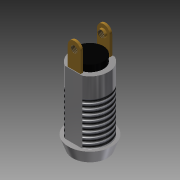
# Autodesk Inventor part: KeySwitchBody
Saved by Autodesk Inventor 2016 (Build 200138000, 138)
## iProperties
Created: 2014-09-27
Part Number: KeySwitchBody
Material: Steel, Alloy
Document SubType Name: Modeling
Designer: Jack
Density: 7.73 g/cm^3
Appearance: Semi-Polished
Mass: 83.2063 g
Surface Area: 38.3023 cm^2
Volume: 10.7641 cm^3
Author: Jack
Autodesk Inventor part; units mm, degrees
ref_plane "YZ Plane" through (0, 0, 0) normal (1, 0, 0) x (0, 1, 0)
ref_plane "XZ Plane" through (0, 0, 0) normal (0, 1, 0) x (-1, 0, 0)
sketch "Sketch1" plane through (0, 0, 0) normal (0, 0, 1) x (1, 0, 0)
  circle A0 centre (0, 0) radius 9.375
  dimension "d0" = 18.75
  constraints: 1 centre point, 1 coincident
  measures "d0" diameter of A0
extrude "Extrusion1" add sketch "Sketch1" along normal blind 32
sketch "Sketch2" plane through (0, 0, 32) normal (0, 0, 1) x (1, 0, 0)
  circle A0 centre (0, 0) radius 9.375 projected
  circle A1 centre (0, 0) radius 6.8
  dimension "d3" = 13.6
  constraints: 1 centre point, 1 coincident
  measures "d3" diameter of A1
extrude "Extrusion2" add sketch "Sketch2" along normal blind 3.3 contours A1
sketch "Sketch3" plane through (0, 0, 32) normal (0, 0, 1) x (1, 0, 0)
  circle A0 centre (0, 0) radius 6.8 projected
  line L0 (-3.25, 8) -> (3.25, 8)
  line L1 (-3.25, -8) -> (3.25, -8)
  line L2 (-3.25, 8) -> (-3.25, 6.8)
  line L3 (-3.25, 6.8) -> (3.25, 6.8)
  line L4 (3.25, 6.8) -> (3.25, 8)
  line L5 (-3.25, -8) -> (-3.25, -6.8)
  line L6 (-3.25, -6.8) -> (3.25, -6.8)
  line L7 (3.25, -6.8) -> (3.25, -8)
  dimension "d6" = 6.5
  dimension "d7" = 6.5
  dimension "d8" = 3.25
  dimension "d9" = 3.25
  dimension "d10" = 1.2
  dimension "d11" = 1.2
  dimension "d12" = 16
  dimension "d13" = 8
  constraints: 16 end point, 4 perpendicular, 2 horizontal, 2 vertical
  measures "d6" distance of L1.start L1.end
  measures "d7" distance of L0.start L0.end
  measures "d8" horizontal distance of A0.centre L1.end
  measures "d9" horizontal distance of L0.end A0.centre
  measures "d10" distance of L0.start L2.end
  measures "d11" distance of L1.start L5.end
  measures "d12" distance between parallel lines of L1 L0
  measures "d13" distance from line of A0.centre L0
extrude "Extrusion3" add sketch "Sketch3" along normal blind 13 contours L6 L7 L1 L5 | L3 L2 L0 L4
sketch "Sketch4" plane through (-3.25, -8, 32) normal (0, -1, 0) x (1, 0, 0)
  line L0 (6.5, 0) -> (6.5, 13) projected
  line L1 (0, 13) -> (6.5, 13) projected
  circle A0 centre (3.25, 9.2) radius 1.7
  point P0 (3.25, -32)
  dimension "d16" = 3.4
  dimension "d17" = 3.25
  dimension "d18" = 3.8
  constraints: 1 centre point
  measures "d16" diameter of A0
  measures "d17" distance from line of L0 A0.centre
  measures "d18" distance from line of L1 A0.centre
extrude "Extrusion4" cut sketch "Sketch4" against normal up to surface (16 mm away)
fillet "Fillet1" radius 3.25 4 edges at (-3.25, -7.4, 45) (3.25, -7.4, 45) (-3.25, 7.4, 45) (3.25, 7.4, 45)
sketch "Sketch5" plane through (-3.25, 6.8, 32) normal (0, -1, 0) x (1, 0, 0)
  circle A0 centre (3.25, 9.2) radius 1.7 projected
  circle A1 centre (3.25, 9.2) radius 1.95
  point P0 (3.25, -32)
  dimension "d22" = 3.9
  constraints: 1 centre point, 1 coincident
  measures "d22" diameter of A1
extrude "Extrusion5" add sketch "Sketch5" along normal blind 1.2
sketch "Sketch6" plane through (0, -6.8, 32) normal (0, 1, 0) x (1, 0, 0)
  circle A0 centre (0, -9.2) radius 1.7 projected
  circle A1 centre (0, -9.2) radius 1.95
  point P0 (0, 32)
  dimension "d25" = 3.9
  constraints: 1 centre point, 1 coincident
  measures "d25" diameter of A1
extrude "Extrusion6" add sketch "Sketch6" along normal blind 1.2
sketch "Sketch7" plane through (0, 0, 0) normal (0, 0, -1) x (-1, 0, 0)
  circle A0 centre (0, 0) radius 9.375 projected
  circle A1 centre (0, 0) radius 10.95
  dimension "d28" = 21.9
  constraints: 1 centre point, 1 coincident
  measures "d28" diameter of A1
ref_plane "Work Plane1" through (0, 0, -6.2) normal (0, 0, -1) x (-1, 0, 0)
sketch "Sketch8" plane through (0, 0, -6.2) normal (0, 0, -1) x (-1, 0, 0)
  circle A0 centre (0, 0) radius 9.375 projected
  circle A1 centre (0, 0) radius 8.75
  dimension "d30" = 17.5
  constraints: 1 centre point, 1 coincident
  measures "d30" diameter of A1
loft "Loft1" add profiles "Sketch7", "Sketch8" contours A0 | A1 / A1
sketch "Sketch9" plane through (0, 0, 32) normal (0, 0, 1) x (1, 0, 0)
  circle A0 centre (0, 0) radius 9.375 projected
  line L0 (-4.359, 8.3) -> (4.359, 8.3)
  line L1 (-4.359, -8.3) -> (4.359, -8.3)
  point P0 (8.3, 4.359)
  point P1 (8.3, -4.359)
  point P2 (-8.3, 4.359)
  point P3 (-8.3, -4.359)
  dimension "d51" = 16.6
  dimension "d52" = 8.3
  constraints: 4 end point, 1 horizontal, 1 parallel, 9 other
  measures "d51" distance between parallel lines of L0 L1
  measures "d52" distance from line of point (0, 0) L1
thread "Thread1" size "M20x2.5" class "6g" standard "ANSI Metric M Profile" length 22
thread "Thread2" size "M20x2.5" class "6g" standard "ANSI Metric M Profile" length 22
thread "Thread3" size "M3.5x0.6" class "6H" standard "ANSI Metric M Profile" length 10
thread "Thread4" size "M3.5x0.6" class "6H" standard "ANSI Metric M Profile" length 10
sketch "Sketch10" plane through (0, 0, -6.2) normal (0, 0, -1) x (-1, 0, 0)
  circle A0 centre (0, 0) radius 8.75 projected
  circle A1 centre (0, 0) radius 4.9
  circle A2 centre (0, 0) radius 3.8
  dimension "d47" = 9.8
  dimension "d48" = 7.6
  constraints: 2 centre point, 2 coincident
  measures "d47" diameter of A1
  measures "d48" diameter of A2
extrude "Extrusion8" cut sketch "Sketch10" against normal blind 6 contours A1
extrude "Extrusion9" cut sketch "Sketch9" against normal up to surface (32 mm away) contours L0 A0 | A0 L1
sketch "Sketch11" plane through (0, 0, -6.2) normal (0, 0, -1) x (-1, 0, 0)
  circle A0 centre (0, 0) radius 3.8 projected
  circle A1 centre (0, 0) radius 8.75 projected
  circle A2 centre (0, 0) radius 4.9 projected
  line L0 (6.1, 0.75) -> (1.7, 0.75)
  line L1 (1.7, 0.75) -> (1.7, -0.75)
  line L2 (1.7, -0.75) -> (6.1, -0.75)
  line L3 (6.1, -0.75) -> (6.1, 0.75)
  circle A3 centre (0, 0) radius 4.9 projected
  line L4 (0.75, -4.8423) -> (0.75, -6.1)
  line L5 (0.75, -6.1) -> (-0.75, -6.1)
  line L6 (-0.75, -6.1) -> (-0.75, -4.8423)
  dimension "d55" = 4.4
  dimension "d56" = 1.5
  dimension "d57" = 1.5
  dimension "d58" = 1.2
  dimension "d59" = 0.75
  dimension "d60" = 1.2
  dimension "d61" = 0.75
  constraints: 14 end point, 4 point on circle, 2 parallel, 2 perpendicular, 2 vertical, 1 horizontal
  measures "d55" distance of L2.end L1.end
  measures "d56" distance of L2.end L0.start
  measures "d57" distance of L4.end L5.end
  measures "d58" distance edge to line of A2 L5
  measures "d59" distance from line of A0.centre L2
  measures "d60" distance edge to line of A2 L3
  measures "d61" distance from line of A0.centre L6
extrude "Extrusion10" cut sketch "Sketch11" against normal up to surface (6 mm away) contours A0 L2 L1 L0 | A0 L0 A2 L2 | L0 L3 L2 A2 | A2 L4 L5 L6 picked at (2.4, 0) picked at (4.1442, -0.4181)
body "Solid1"
